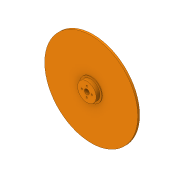
# Autodesk Inventor part: P_foot_001
Saved by Autodesk Inventor 2016 (Build 200138000, 138)
## iProperties
Created: 2016-02-23
Part Number: P_foot_001
Material: PC/ABS Plastic
Document SubType Name: Modeling
Designer: Mateusz
Density: 0.357273 g/cm^3
Appearance: Orange
Author: Mateusz
Autodesk Inventor part; units mm, degrees
ref_plane "YZ Plane" through (0, 0, 0) normal (1, 0, 0) x (0, 1, 0)
ref_plane "XZ Plane" through (0, 0, 0) normal (0, 1, 0) x (-1, 0, 0)
ref_plane "XY Plane" through (0, 0, 0) normal (0, 0, 1) x (1, 0, 0)
derived "skeleton.ipt"
sketch "Sketch2" plane through (0, 0, 0) normal (0, 0, 1) x (1, 0, 0)
  circle A0 centre (0, 0) radius 75
  dimension "d1" = 150
  constraints: 1 centre point, 1 coincident
  measures "d1" diameter of A0
extrude "Extrusion1" add sketch "Sketch2" along normal blind 3
sketch "Sketch4" plane through (0, 0, 3) normal (0, 0, 1) x (1, 0, 0)
  circle A0 centre (0, 0) radius 18
  dimension "d11" = 36
  constraints: 1 centre point, 1 coincident
  measures "d11" diameter of A0
extrude "Extrusion2" add sketch "Sketch4" along normal blind 1
sketch "Sketch6" plane through (0, 0, 4) normal (0, 0, 1) x (1, 0, 0)
  circle A0 centre (0, 0) radius 15
  dimension "d18" = 30
  constraints: 1 centre point, 1 coincident
  measures "d18" diameter of A0
extrude "Extrusion4" add sketch "Sketch6" along normal blind 6
sketch "Sketch7" plane through (0, 0, 10) normal (0, 0, 1) x (1, 0, 0)
  circle A0 centre (0, 0) radius 3.1 projected
  circle A1 centre (-0.2026, -7.9974) radius 1.25 projected
  circle A2 centre (-7.9974, 0.2026) radius 1.25 projected
  circle A3 centre (0.2026, 7.9974) radius 1.25 projected
  circle A4 centre (-5.4982, 0.1393) radius 0.75 projected
  circle A5 centre (2.6285, -4.8312) radius 0.75 projected
  circle A6 centre (2.8697, 4.692) radius 0.75 projected
  arc A7 (9.2286, 0.0136) -> (9.2161, -0.4807) centre (7.9974, -0.2026) ccw projected
  line L0 (9.2161, -0.4807) -> (10.9874, -0.5256) projected
  arc A8 (-10.9653, -0.8726) -> (10.9874, -0.5256) centre (0, 0) ccw projected
  line L1 (-10.9653, -0.8726) -> (-10.6257, -0.8812) projected
  line L2 (-10.6257, -0.8812) -> (-10.6181, -0.5813) projected
  line L3 (-10.6181, -0.5813) -> (-10.9851, -0.572) projected
  arc A9 (-10.9421, 1.1274) -> (-10.9851, -0.572) centre (0, 0) ccw projected
  line L4 (-10.9421, 1.1274) -> (-10.5751, 1.1181) projected
  line L5 (-10.5751, 1.1181) -> (-10.5675, 1.418) projected
  line L6 (-10.5675, 1.418) -> (-10.9071, 1.4266) projected
  arc A10 (11, -0.0313) -> (-10.9071, 1.4266) centre (0, 0) ccw projected
  line L7 (11, -0.0313) -> (9.2286, 0.0136) projected
  point P0 (0, 0)
  constraints: 4 coincident
hole "Hole2" at (7.9974, -0.2026, 10) at (0.2026, 7.9974, 10) at (-7.9974, 0.2026, 10) at (-0.2026, -7.9974, 10) direction (0, 0, -1) diameter 2.6 end through all
sketch "Sketch8" plane through (0, 0, 0) normal (0, 0, -1) x (-1, 0, 0)
  circle A0 centre (0, 0) radius 75 projected
  circle A1 centre (0, 0) radius 4
  point P0 (0, 0)
  dimension "d28" = 8
  constraints: 1 centre point, 1 coincident
  measures "d28" diameter of A1
extrude "Extrusion5" cut sketch "Sketch8" against normal up to next contours A1
equation "\"d1\" = foot_length"
equation "\"foot_length\" = 150"
body "Solid1"
